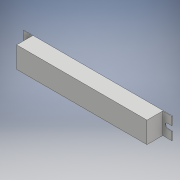
# Autodesk Inventor part: Balastro
Saved by Autodesk Inventor 2017 (Build 210142000, 142)
## iProperties
Created: 2021-01-04
Part Number: Balastro
Material: Generic
Document SubType Name: Modeling
Designer: USUARIO
Density: 1 g/cm^3
Appearance: Default
Author: USUARIO
Autodesk Inventor part; units mm, degrees
ref_plane "YZ Plane" through (0, 0, 0) normal (1, 0, 0) x (0, 1, 0)
ref_plane "XZ Plane" through (0, 0, 0) normal (0, 1, 0) x (-1, 0, 0)
ref_plane "XY Plane" through (0, 0, 0) normal (0, 0, 1) x (1, 0, 0)
sketch "Sketch1" plane through (0, 0, 0) normal (0, 1, 0) x (-1, 0, 0)
  line L0 (0, 0) -> (215, 0)
  line L1 (215, 0) -> (215, -35)
  line L2 (215, -35) -> (0, -35)
  line L3 (0, -35) -> (0, 0)
  dimension "d0" = 215
  dimension "d1" = 35
  constraints: 8 end point, 2 parallel, 1 horizontal, 1 perpendicular
  measures "d0" distance of L1.end L2.end
  measures "d1" distance of L0.end L1.end
extrude "Extrusion1" add sketch "Sketch1" along normal blind 27
sketch "Sketch2" plane through (0, 27, 0) normal (0, 1, 0) x (1, 0, 0)
  line L0 (0, 0) -> (15, 0)
  line L1 (15, 0) -> (15, 35)
  line L2 (15, 35) -> (0, 35)
  line L3 (0, 35) -> (0, 0)
  line L4 (-215, 35) -> (-215, 0) projected
  line L5 (-215, 0) -> (-230, 0)
  line L6 (-230, 0) -> (-230, 35)
  line L7 (-230, 35) -> (-215, 35)
  line L8 (-215, 35) -> (-215, 0)
  dimension "d4" = 15
  dimension "d5" = 35
  dimension "d6" = 15
  dimension "d7" = 35
  constraints: 16 end point, 4 parallel, 2 horizontal, 2 perpendicular
  measures "d4" distance of L2.end L1.end
  measures "d5" distance of L1.end L0.end
  measures "d6" distance of L6.end L7.end
  measures "d7" distance of L5.end L6.end
extrude "Extrusion2" add sketch "Sketch2" against normal blind 1
sketch "Sketch3" plane through (0, 27, 0) normal (0, 1, 0) x (1, 0, 0)
  line L0 (15, 13.5) -> (8, 13.5)
  line L1 (4, 17.5) -> (4, 17.5)
  line L2 (8, 21.5) -> (15, 21.5)
  line L3 (15, 21.5) -> (15, 13.5)
  line L4 (15, 35) -> (-230, 35) projected
  line L5 (15, 0) -> (15, 35) projected
  line L6 (-230, 13.5) -> (-223, 13.5)
  line L7 (-219, 17.5) -> (-219, 17.5)
  line L8 (-223, 21.5) -> (-230, 21.5)
  line L9 (-230, 21.5) -> (-230, 13.5)
  line L10 (15, 0) -> (-230, 0) projected
  arc A0 (-223, 13.5) -> (-219, 17.5) centre (-223, 17.5) ccw
  arc A1 (-219, 17.5) -> (-223, 21.5) centre (-223, 17.5) ccw
  line L11 (-230, 0) -> (-230, 35) projected
  arc A2 (4, 17.5) -> (8, 13.5) centre (8, 17.5) ccw
  arc A3 (8, 21.5) -> (4, 17.5) centre (8, 17.5) ccw
  point P0 (0, 0)
  point P1 (4, 21.5)
  point P2 (4, 13.5)
  point P3 (-219, 21.5)
  point P4 (-219, 13.5)
  dimension "d10" = 11
  dimension "d11" = 8
  dimension "d12" = 13.5
  dimension "d13" = 0
  dimension "d14" = 11
  dimension "d15" = 8
  dimension "d16" = 13.5
  dimension "d17" = 4
  dimension "d18" = 4
  dimension "d19" = 0
  dimension "d20" = 4
  constraints: 16 end point, 8 point on circle, 8 point on line, 8 tangent, 4 centre point, 4 parallel, 2 horizontal, 2 perpendicular, 1 concentric
  measures "d10" distance of point (4, 21.5) L2.end
  measures "d11" distance of point (4, 13.5) point (4, 21.5)
  measures "d12" distance between parallel lines of L4 L2
  measures "d13" distance between parallel lines of L5 L3
  measures "d14" distance of L8.end point (-219, 21.5)
  measures "d15" distance of point (-219, 21.5) point (-219, 13.5)
  measures "d16" distance between parallel lines of L10 L6
  measures "d17" radius of A0
  measures "d18" radius of A1
  measures "d19" distance between parallel lines of L11 L9
  measures "d20" radius of A2
extrude "Extrusion3" cut sketch "Sketch3" against normal blind 1 contours L0 A2 A3 L2 L3 | L9 L8 A1 A0 L6
body "Solid1"
